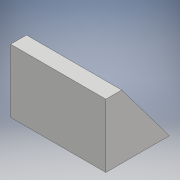
# Autodesk Inventor part: 9
Saved by Autodesk Inventor 2017 (Build 210142000, 142)
## iProperties
Part Number: 9
Material: 一般
Document SubType Name: Modeling
Designer: Brian
Density: 1 g/cm^3
Appearance: 預設
Author: Brian
Autodesk Inventor part; units mm, degrees
ref_plane "YZ Plane" through (0, 0, 0) normal (1, 0, 0) x (0, 1, 0)
ref_plane "XZ Plane" through (0, 0, 0) normal (0, 1, 0) x (-1, 0, 0)
ref_plane "XY Plane" through (0, 0, 0) normal (0, 0, 1) x (1, 0, 0)
sketch "草圖1" plane through (0, 0, 0) normal (0, 1, 0) x (-1, 0, 0)
  line L0 (0, 0) -> (-60, 0)
  line L1 (-60, 0) -> (-60, -40)
  line L2 (-60, -40) -> (0, -40)
  line L3 (0, -40) -> (0, 0)
  dimension "d0" = 40
  dimension "d1" = 60
  constraints: 8 end point, 2 parallel, 1 horizontal, 1 perpendicular
  measures "d0" distance of L2.end L0.start
  measures "d1" distance of L1.end L2.end
extrude "擠出1" add sketch "草圖1" along normal blind 10
sketch "草圖2" plane through (0, 10, 0) normal (0, 1, 0) x (1, 0, 0)
  line L0 (60, 40) -> (0, 40) projected
  line L1 (0, 40) -> (20, 40)
  line L2 (20, 40) -> (20, 0)
  line L3 (20, 0) -> (0, 0)
  line L4 (0, 0) -> (0, 40)
  line L5 (60, 0) -> (60, 40) projected
  line L6 (0, 0) -> (60, 0) projected
  line L7 (60, 40) -> (40, 40)
  line L8 (40, 40) -> (40, 0)
  line L9 (40, 0) -> (60, 0)
  line L10 (60, 0) -> (60, 40)
  dimension "d4" = 40
  dimension "d5" = 20
  dimension "d6" = 20
  constraints: 16 end point, 4 parallel, 2 horizontal, 2 perpendicular, 1 point on line
  measures "d4" distance of L1.end L2.end
  measures "d5" distance between parallel lines of L8 L2
  measures "d6" distance between parallel lines of L5 L8
extrude "擠出2" add sketch "草圖2" along normal blind 30 contours L5 L6 L8 L0 | L2 L3 L4 L0
sketch "草圖3" plane through (60, 0, 0) normal (1, 0, 0) x (0, 0, -1)
  line L0 (40, 40) -> (0, 40) projected
  line L1 (40, 40) -> (0, 10)
  line L2 (0, 10) -> (0, 40)
  line L3 (40, 0) -> (40, 40) projected
  line L4 (0, 40) -> (40, 40)
  point P0 (0, 0)
  dimension "d9" = 30
  constraints: 6 end point, 2 perpendicular
  measures "d9" distance of L1.end L0.end
extrude "擠出3" cut sketch "草圖3" against normal through all
sketch "草圖4" plane through (0, 10, 0) normal (0, 1, 0) x (1, 0, 0)
  line L0 (40, 40) -> (20, 40) projected
  line L1 (20, 40) -> (10, 0)
  line L2 (0, 0) -> (60, 0) projected
  line L3 (40, 40) -> (50, 0)
  line L4 (20, 40) -> (20, 0) projected
  line L5 (20, 0) -> (40, 0) projected
  line L6 (40, 0) -> (40, 40) projected
  line L7 (40, 40) -> (20, 40) projected
  line L8 (20, 40) -> (40, 40)
  line L9 (60, 40) -> (0, 40) projected
  line L10 (10, 0) -> (50, 0)
  dimension "d12" = 10
  dimension "d13" = 10
  constraints: 8 end point, 2 collinear, 1 horizontal alignment, 1 point on line
  measures "d12" horizontal distance of L0.start L3.end
  measures "d13" horizontal distance of L0.end L1.end
extrude "擠出4" cut sketch "草圖4" along normal through all
